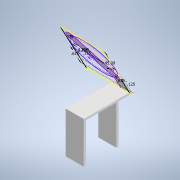
# Autodesk Inventor part: Motor Mount
Saved by Autodesk Inventor 2021 (Build 250183000, 183)
## iProperties
Created: 2020-12-19
Part Number: Motor Mount
Material: Generic
Document SubType Name: Modeling
Designer: Ramsey
Density: 1 g/cm^3
Appearance: Default
Author: Ramsey
Autodesk Inventor part; units mm, degrees
ref_plane "YZ Plane" through (0, 0, 0) normal (1, 0, 0) x (0, 1, 0)
ref_plane "XZ Plane" through (0, 0, 0) normal (0, 1, 0) x (-1, 0, 0)
ref_plane "XY Plane" through (0, 0, 0) normal (0, 0, 1) x (1, 0, 0)
sketch "Sketch1" plane through (0, 0, 0) normal (1, 0, 0) x (0, 1, 0)
  line L0 (6.6158, 26.6317) -> (-24.673, 26.6317)
  line L1 (6.6158, 0.5934) -> (6.6158, 26.6317)
  line L2 (5.0158, 25.0317) -> (-24.673, 25.0317)
  line L3 (-24.673, 1.8624) -> (5.0158, 1.8624)
  line L4 (5.0158, 1.8624) -> (5.0158, 25.0317)
  line L5 (-24.673, 26.6317) -> (-24.673, 25.0317)
  line L6 (-24.673, 1.8624) -> (-24.673, 0.1625)
  line L7 (-24.6286, 24.997) -> (4.9714, 24.997) construction
  line L8 (4.9714, 24.997) -> (4.9714, 1.897) construction
  line L9 (4.9714, 1.897) -> (-24.6286, 1.897) construction
  line L10 (-24.6286, 1.897) -> (-24.6286, 24.997) construction
  line L11 (-24.6286, 1.897) -> (-24.6286, 1.8624) construction
  line L12 (-24.6286, 24.997) -> (-24.6286, 25.0317) construction
  line L13 (4.9714, 2.1686) -> (16.2714, -18.903) construction
  line L14 (4.0247, -13.8964) -> (20.8987, -4.8474)
  line L15 (5.0283, -10.6206) -> (44.2273, 10.4005)
  line L16 (5.0283, -10.6206) -> (5.0283, 0.1625)
  line L17 (6.6158, 0.5934) -> (6.6158, -7.968)
  line L18 (6.6158, -7.968) -> (43.477, 11.7995)
  line L19 (43.477, 11.7995) -> (44.2273, 10.4005)
  line L20 (-24.673, 0.1625) -> (5.0283, 0.1625)
  line L21 (6.6158, 13.8186) -> (15.6898, -3.1019) construction
  point P0 (0, 0)
  dimension "d2" = 1.6
  dimension "d3" = 23.1693
  dimension "d5" = 29.6888
  dimension "d6" = 29.6
  dimension "d7" = 23.1
  dimension "d8" = 0.0444
  dimension "d9" = 11.3
  dimension "d10" = 20.8
  dimension "d11" = 10.2
  dimension "d15" = 1.5875
  dimension "d22" = 4
  dimension "d23" = 1.5875
  dimension "d28" = 19.2
  constraints: 44 end point, 8 perpendicular, 7 parallel, 6 point on line, 3 collinear, 2 horizontal, 2 vertical, 1 other
  measures "d2" distance between parallel lines of L1 L4
  measures "d3" distance of L3.end L2.start
  measures "d5" distance of L2.start L2.end
  measures "d6" distance of L7.start L7.end
  measures "d7" distance of L9.end L7.start
  measures "d8" distance between parallel lines of L4 L8
  measures "d9" distance from line of L8 L13.end
  measures "d10" distance from line of L13.end L9
  measures "d11" distance from line of L13.end L14
  measures "d15" distance between parallel lines of L17 L16
  measures "d22" distance between parallel lines of L14 L18
  measures "d23" distance of L18.end L15.end
  measures "d28" distance of L21.start L21.end
extrude "Extrusion1" add sketch "Sketch1" along normal blind 32.6644
sketch "Sketch2" plane through (0, 6.6158, -7.968) normal (0, -0.4726007, 0.8812767) x (1, 0, 0)
  circle A0 centre (17.209, 24.6192) radius 16.4
  circle A1 centre (28.8056, 13.0227) radius 1
  circle A2 centre (5.6125, 36.2158) radius 1
  line L0 (28.8056, 13.0227) -> (5.6125, 36.2158) construction
  line L1 (0, 41.827) -> (32.6644, 41.827) projected
  line L2 (0, 3.3414) -> (38.1, 3.3414) construction
  line L3 (0, 41.827) -> (0, 0) construction
  circle A3 centre (11.5522, 18.9624) radius 1.4362 construction
  line L4 (11.5522, 18.9624) -> (17.209, 24.6192) construction
  line L5 (0, 10.2963) -> (32.6644, 10.2963) construction
  line L6 (32.6644, 41.827) -> (32.6644, 0) construction
  circle A4 centre (17.209, 24.6192) radius 13.95 construction
  line L7 (28.8056, 13.0227) -> (5.6125, 36.2158) construction
  line L8 (31.7345, 15.4934) -> (8.3123, 38.9155)
  line L9 (2.9127, 33.516) -> (26.1058, 10.3229)
  arc A5 (26.1058, 10.3229) -> (26.1326, 10.2963) centre (28.8056, 13.0227) ccw
  arc A6 (8.3123, 38.9155) -> (2.9127, 33.516) centre (5.6125, 36.2158) ccw
  line L10 (32.6644, 13.2483) -> (32.6644, 0)
  line L11 (0, 0) -> (32.6644, 0) projected
  line L12 (26.1326, 10.2963) -> (26.1326, 0)
  arc A7 (32.6644, 13.2483) -> (31.7345, 15.4934) centre (29.4894, 13.2483) ccw
  line L13 (0, 0) -> (0, 41.827)
  line L14 (32.6644, -2.6527) -> (32.6644, 41.827) projected
  arc A8 (17.872, 18.5567) -> (11.1465, 25.2822) centre (11.4175, 18.8277) ccw
  point P0 (0, -2.0647)
  point P1 (0, 3.3414)
  point P2 (0, 10.2963)
  point P3 (31.1867, 16.0411)
  point P4 (32.6644, 19.1336)
  point P5 (32.6644, 13.2483)
  point P6 (15.9856, 23.3958)
  dimension "d16" = 32.8
  dimension "d17" = 2
  dimension "d18" = 2
  dimension "d19" = 45
  dimension "d26" = 8
  dimension "d27" = 15.621
  dimension "d29" = 27.9
  dimension "d30" = 3.175
  constraints: 22 end point, 11 point on circle, 9 centre point, 6 point on line, 6 tangent, 4 perpendicular, 2 midpoint, 2 parallel, 1 coincident, 1 collinear, 1 vertical, 2 other
  measures "d16" diameter of A0
  measures "d17" diameter of A1
  measures "d18" diameter of A2
  measures "d19" angle of L1 L0
  measures "d26" distance of L4.start L4.end
  measures "d27" distance from line of L2 L4.start
  measures "d29" diameter of A4
  measures "d30" radius of A7
extrude "Extrusion2" cut sketch "Sketch2" against normal blind 25.4 contours A2 A0 | A0 A2 | A1 A0 | A0 A1
extrude "Extrusion3" cut sketch "Sketch2" against normal blind 25.4 contours L14 A0 L8 | A0 L8 A6 L9 A5 L12 L11 L13 L1 L14 | L14 A7 L8 A0 | L9 A0 | A8 L9
sketch "Sketch5" plane through (0, 0, 0) normal (-1, 0, 0) x (0, 0, 1)
  line L0 (-7.968, 6.6158) -> (-9.367, 7.3661) projected
  line L1 (-10.6206, 5.0283) -> (-9.367, 7.3661) projected
  line L2 (0.1625, 5.0283) -> (-10.6206, 5.0283) projected
  line L3 (0.1625, -24.673) -> (0.1625, 5.0283) projected
  line L4 (1.8624, -24.673) -> (0.1625, -24.673) projected
  line L5 (1.8624, 5.0158) -> (1.8624, -24.673) projected
  line L6 (25.0317, 5.0158) -> (1.8624, 5.0158) projected
  line L7 (25.0317, -24.673) -> (25.0317, 5.0158) projected
  line L8 (26.6317, -24.673) -> (25.0317, -24.673) projected
  line L9 (26.6317, 6.6158) -> (26.6317, -24.673) projected
  line L10 (-7.968, 6.6158) -> (26.6317, 6.6158) projected
  point P0 (0, 0)
extrude "Extrusion4" cut sketch "Sketch5" against normal blind 19.05
body "Solid1"
